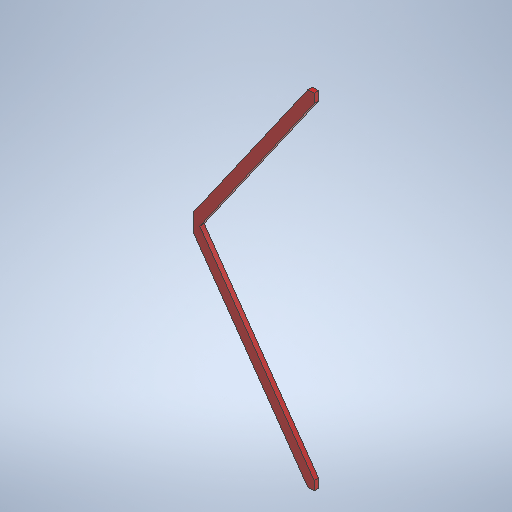
# Autodesk Inventor part: side2
Saved by Autodesk Inventor 2025.1 (Build 291241020, 241B)
## iProperties
Created: 2024-09-20
Part Number: side2
Material: Generic
Document SubType Name: Modeling
Designer: User
Density: 1 g/cm^3
Appearance: Default
Author: User
Autodesk Inventor part; units mm, degrees
ref_plane "YZ Plane" through (0, 0, 0) normal (1, 0, 0) x (0, 1, 0)
ref_plane "XZ Plane" through (0, 0, 0) normal (0, 1, 0) x (-1, 0, 0)
ref_plane "XY Plane" through (0, 0, 0) normal (0, 0, 1) x (1, 0, 0)
sketch "Sketch1" plane through (0, 0, 0) normal (0, 0, 1) x (1, 0, 0)
  line L0 (88.9, 0) -> (88.9, 3048) projected
  line L1 (1130.3, 38.1) -> (88.9, 38.1) projected
  line L2 (1130.3, 0) -> (1130.3, 3048) projected
  line L3 (88.9, 3009.9) -> (1130.3, 3009.9) projected
  line L4 (1130.3, 115.5482) -> (143.1799, 1524)
  line L5 (143.1799, 1524) -> (1130.3, 2932.4518)
  line L6 (1076.0201, 3009.9) -> (88.9, 1601.4482)
  line L7 (88.9, 1446.5518) -> (1076.0201, 38.1)
  line L8 (1076.0201, 38.1) -> (1130.3, 38.1)
  line L9 (1130.3, 38.1) -> (1130.3, 115.5482)
  line L10 (1130.3, 2932.4518) -> (1130.3, 3009.9)
  line L11 (1076.0201, 3009.9) -> (1130.3, 3009.9)
  line L12 (88.9, 1601.4482) -> (88.9, 1446.5518)
  line L13 (88.9, 1446.5518) -> (88.9, 1601.4482)
  point P0 (0, 0)
  constraints: 20 end point, 6 point on line, 4 collinear, 2 parallel, 2 perpendicular
extrude "Extrusion1" add sketch "Sketch1" against normal blind 38.1 contours L0 L6 L3 L2 L5 L4 L1 L7
body "Solid1"
